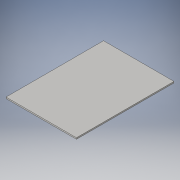
# Autodesk Inventor part: KrackenPlate1
Saved by Autodesk Inventor 2016 (Build 200138000, 138)
## iProperties
Created: 2015-09-01
Part Number: KrackenPlate1
Material: Generic
Document SubType Name: Modeling
Designer: Tim
Density: 1 g/cm^3
Appearance: Default
Author: Tim
Autodesk Inventor part; units mm, degrees
ref_plane "YZ Plane" through (0, 0, 0) normal (1, 0, 0) x (0, 1, 0)
ref_plane "XZ Plane" through (0, 0, 0) normal (0, 1, 0) x (-1, 0, 0)
ref_plane "XY Plane" through (0, 0, 0) normal (0, 0, 1) x (1, 0, 0)
sketch "Sketch1" plane through (0, 0, 0) normal (0, 1, 0) x (-1, 0, 0)
  line L0 (104, -144) -> (-104, -144)
  line L1 (-104, -144) -> (-104, 144)
  line L2 (-104, 144) -> (104, 144)
  line L3 (104, 144) -> (104, -144)
  line L4 (104, -144) -> (-104, 144) construction
  line L5 (-104, -144) -> (104, 144) construction
  point P0 (0, 0)
  dimension "d0" = 208
  dimension "d1" = 288
  constraints: 12 end point, 2 midpoint, 2 parallel, 1 horizontal, 1 perpendicular
  measures "d0" distance of L1.end L2.end
  measures "d1" distance of L2.end L0.start
extrude "Extrusion3" add sketch "Sketch1" along normal blind 4
body "Solid3"
